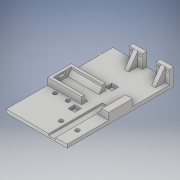
# Autodesk Inventor part: Elevator Slide Top
Saved by Autodesk Inventor 2018 (Build 220112000, 112)
## iProperties
Created: 2017-10-26
Part Number: Elevator Slide Top
Material: Generic
Document SubType Name: Modeling
Designer: thompson.nathaniel
Density: 1 g/cm^3
Appearance: Default
Author: thompson.nathaniel
Autodesk Inventor part; units mm, degrees
ref_plane "YZ Plane" through (0, 0, 0) normal (1, 0, 0) x (0, 1, 0)
ref_plane "XZ Plane" through (0, 0, 0) normal (0, 1, 0) x (-1, 0, 0)
ref_plane "XY Plane" through (0, 0, 0) normal (0, 0, 1) x (1, 0, 0)
sketch "Sketch1" plane through (0, 0, 0) normal (0, 1, 0) x (-1, 0, 0)
  line L0 (0, 0) -> (-114.3, 0)
  line L1 (-114.3, 0) -> (-114.3, 152.4)
  line L2 (-114.3, 152.4) -> (0, 152.4)
  line L3 (0, 152.4) -> (0, 0)
  line L4 (-57.15, 34.925) -> (-69.85, 34.925)
  line L5 (-69.85, 34.925) -> (-69.85, 47.625)
  line L6 (-69.85, 47.625) -> (-57.15, 47.625)
  line L7 (-57.15, 47.625) -> (-57.15, 34.925)
  line L8 (-57.15, 104.775) -> (-69.85, 104.775)
  line L9 (-69.85, 104.775) -> (-69.85, 117.475)
  line L10 (-69.85, 117.475) -> (-57.15, 117.475)
  line L11 (-57.15, 117.475) -> (-57.15, 104.775)
  dimension "d0" = 152.4
  dimension "d1" = 114.3
  dimension "d2" = 12.7
  dimension "d3" = 12.7
  dimension "d4" = 12.7
  dimension "d5" = 12.7
  dimension "d6" = 34.925
  dimension "d7" = 34.925
  dimension "d8" = 44.45
  dimension "d9" = 44.45
  constraints: 24 end point, 6 parallel, 3 horizontal, 3 perpendicular
  measures "d0" distance of L2.end L0.start
  measures "d1" distance of L0.start L0.end
  measures "d2" distance of L4.start L4.end
  measures "d3" distance of L8.start L8.end
  measures "d4" distance of L8.end L9.end
  measures "d5" distance of L4.end L5.end
  measures "d6" distance between parallel lines of L0 L4
  measures "d7" distance between parallel lines of L2 L10
  measures "d8" distance between parallel lines of L1 L5
  measures "d9" distance between parallel lines of L1 L9
extrude "Extrusion1" add sketch "Sketch1" along normal blind 10.16
sketch "Sketch2" plane through (0, 0, 0) normal (-1, 0, 0) x (0, 0, 1)
  line L0 (0, 10.16) -> (152.4, 10.16) projected
  line L1 (53.975, 10.16) -> (98.425, 10.16)
  line L2 (98.425, 10.16) -> (98.425, 22.86)
  line L3 (98.425, 22.86) -> (93.345, 22.86)
  line L4 (93.345, 22.86) -> (93.345, 19.05)
  line L5 (93.345, 19.05) -> (86.614, 10.16)
  line L6 (86.614, 10.16) -> (76.2, 10.16)
  line L7 (65.786, 10.16) -> (59.055, 19.05)
  line L8 (59.055, 19.05) -> (59.055, 22.86)
  line L9 (59.055, 22.86) -> (53.975, 22.86)
  line L10 (53.975, 22.86) -> (53.975, 10.16)
  line L11 (0, 0) -> (0, 10.16) projected
  dimension "d12" = 0
  dimension "d13" = 20.828
  dimension "d14" = 44.45
  dimension "d15" = 3.81
  dimension "d16" = 3.81
  dimension "d17" = 12.7
  dimension "d18" = 12.7
  dimension "d19" = 5.08
  dimension "d20" = 5.08
  dimension "d21" = 11.811
  dimension "d24" = 53.975
  constraints: 20 end point, 5 point on line, 4 perpendicular, 2 vertical, 1 midpoint
  measures "d12" distance from line of L1.start L10
  measures "d13" distance of L5.end L7.start
  measures "d14" distance between parallel lines of L2 L10
  measures "d15" distance of L8.end L7.end
  measures "d16" distance of L3.end L4.end
  measures "d17" distance of L9.end L10.end
  measures "d18" distance of L1.end L2.end
  measures "d19" distance of L8.end L9.end
  measures "d20" distance of L2.end L3.end
  measures "d21" distance from line of L7.start L10
  measures "d24" distance between parallel lines of L11 L10
extrude "Extrusion2" add sketch "Sketch2" against normal blind 63.5
sketch "Sketch4" plane through (0, 10.16, 0) normal (0, 1, 0) x (1, 0, 0)
  circle A0 centre (20.32, -47.625) radius 3.81
  circle A1 centre (44.45, -47.625) radius 3.81
  circle A2 centre (20.32, -104.775) radius 3.81
  circle A3 centre (44.45, -104.775) radius 3.81
  line L0 (0, -53.975) -> (63.5, -53.975) projected
  line L1 (63.5, -98.425) -> (0, -98.425) projected
  line L2 (0, -98.425) -> (0, -152.4) projected
  line L3 (0, 0) -> (0, -53.975) projected
  dimension "d28" = 7.62
  dimension "d29" = 7.62
  dimension "d30" = 7.62
  dimension "d31" = 7.62
  dimension "d32" = 6.35
  dimension "d33" = 6.35
  dimension "d34" = 6.35
  dimension "d35" = 6.35
  dimension "d36" = 20.32
  dimension "d37" = 44.45
  dimension "d38" = 20.32
  dimension "d39" = 44.45
  constraints: 4 centre point
  measures "d28" diameter of A0
  measures "d29" diameter of A1
  measures "d30" diameter of A2
  measures "d31" diameter of A3
  measures "d32" distance from line of L0 A0.centre
  measures "d33" distance from line of L0 A1.centre
  measures "d34" distance from line of L1 A3.centre
  measures "d35" distance from line of L1 A2.centre
  measures "d36" distance from line of L2 A2.centre
  measures "d37" distance from line of L2 A3.centre
  measures "d38" distance from line of L3 A0.centre
  measures "d39" distance from line of L3 A1.centre
extrude "Extrusion4" cut sketch "Sketch4" against normal blind 10.16
sketch "Sketch5" plane through (0, 0, 152.4) normal (0, 0, 1) x (1, 0, 0)
  line L0 (0, 0) -> (114.3, 0) projected
  line L1 (0, 10.16) -> (114.3, 10.16)
  line L2 (114.3, 10.16) -> (114.3, 0)
  line L3 (114.3, 0) -> (0, 0)
  line L4 (0, 0) -> (0, 10.16)
  constraints: 8 end point, 2 parallel, 1 horizontal, 1 perpendicular
extrude "Extrusion5" add sketch "Sketch5" along normal blind 25.4
sketch "Sketch6" plane through (114.3, 0, 0) normal (0, 0, -1) x (-1, 0, 0)
  line L0 (0, 10.16) -> (114.3, 10.16) projected
  line L1 (114.3, 0) -> (0, 0) projected
  line L2 (0, 10.16) -> (114.3, 10.16)
  line L3 (114.3, 10.16) -> (114.3, 0)
  line L4 (114.3, 0) -> (0, 0)
  line L5 (0, 0) -> (0, 10.16)
  constraints: 8 end point, 2 parallel, 1 horizontal, 1 perpendicular
extrude "Extrusion6" add sketch "Sketch6" along normal blind 25.4
sketch "Sketch7" plane through (0, 10.16, 0) normal (0, 1, 0) x (1, 0, 0)
  line L0 (114.3, 25.4) -> (114.3, -177.8) projected
  line L1 (114.3, -98.425) -> (101.6, -98.425)
  line L2 (101.6, -98.425) -> (101.6, -53.975)
  line L3 (101.6, -53.975) -> (114.3, -53.975)
  line L4 (114.3, -53.975) -> (114.3, -98.425)
  line L5 (0, -98.425) -> (63.5, -98.425) projected
  line L6 (0, -53.975) -> (63.5, -53.975) projected
  point P0 (0, 0)
  dimension "d46" = 0
  dimension "d47" = 0
  dimension "d48" = 12.7
  constraints: 8 end point, 2 parallel, 1 horizontal, 1 perpendicular, 1 point on line
  measures "d46" distance between parallel lines of L1 L5
  measures "d47" distance between parallel lines of L3 L6
  measures "d48" distance between parallel lines of L0 L2
extrude "Extrusion7" add sketch "Sketch7" along normal blind 12.7
sketch "Sketch8" plane through (0, 10.16, 0) normal (0, 1, 0) x (1, 0, 0)
  line L0 (114.3, -177.8) -> (0, -177.8) projected
  line L1 (80.01, -177.8) -> (92.71, -177.8)
  line L2 (92.71, -177.8) -> (92.71, -76.2)
  line L3 (92.71, -76.2) -> (80.01, -76.2)
  line L4 (80.01, -76.2) -> (80.01, -177.8)
  line L5 (101.6, -98.425) -> (101.6, -53.975) projected
  point P0 (0, 0)
  dimension "d51" = 8.89
  dimension "d52" = 12.7
  dimension "d53" = 101.6
  constraints: 8 end point, 2 parallel, 1 horizontal, 1 perpendicular, 1 point on line
  measures "d51" distance between parallel lines of L5 L2
  measures "d52" distance between parallel lines of L4 L2
  measures "d53" distance between parallel lines of L0 L3
extrude "Extrusion8" cut sketch "Sketch8" against normal blind 3.175
sketch "Sketch9" plane through (0, 0, 0) normal (0, -1, 0) x (1, 0, 0)
  line L0 (0, 177.8) -> (0, -25.4) projected
  line L1 (114.3, 177.8) -> (92.71, 177.8) projected
  line L2 (0, -25.4) -> (114.3, -25.4)
  line L3 (114.3, -25.4) -> (114.3, 177.8)
  line L4 (114.3, 177.8) -> (0, 177.8)
  line L5 (0, 177.8) -> (0, -25.4)
  point P0 (0, 0)
  constraints: 8 end point, 2 parallel, 1 horizontal, 1 perpendicular
extrude "Extrusion9" cut sketch "Sketch9" against normal blind 3.81
sketch "Sketch10" plane through (0, 10.16, 0) normal (0, 1, 0) x (1, 0, 0)
  circle A0 centre (71.12, -144.145) radius 3.81
  circle A1 centre (101.6, -144.145) radius 3.81
  line L0 (0, -93.345) -> (63.5, -93.345) projected
  line L1 (92.71, -76.2) -> (92.71, -177.8) projected
  line L2 (80.01, -177.8) -> (80.01, -76.2) projected
  point P0 (0, 0)
  dimension "d58" = 50.8
  dimension "d59" = 50.8
  dimension "d60" = 7.62
  dimension "d61" = 7.62
  dimension "d68" = 8.89
  dimension "d69" = 8.89
  constraints: 2 centre point
  measures "d58" distance from line of L0 A0.centre
  measures "d59" distance from line of L0 A1.centre
  measures "d60" diameter of A1
  measures "d61" diameter of A0
  measures "d68" distance from line of L1 A1.centre
  measures "d69" distance from line of L2 A0.centre
extrude "Extrusion10" cut sketch "Sketch10" against normal blind 25.4
sketch "Sketch11" plane through (0, 0, 177.8) normal (0, 0, 1) x (1, 0, 0)
  line L0 (0, 10.16) -> (0, 19.05) projected
  line L1 (0, 10.16) -> (114.3, 10.16)
  line L2 (114.3, 10.16) -> (114.3, 3.81)
  line L3 (114.3, 3.81) -> (0, 3.81)
  line L4 (0, 3.81) -> (0, 10.16)
  point P0 (0, 0)
  constraints: 8 end point, 2 parallel, 1 horizontal, 1 perpendicular
extrude "Extrusion11" cut sketch "Sketch11" against normal blind 1.397
sketch "Sketch12" plane through (114.3, 0, -25.4) normal (0, 0, -1) x (-1, 0, 0)
  line L0 (114.3, 19.05) -> (114.3, 10.16) projected
  line L1 (0, 10.16) -> (0, 3.81) projected
  line L2 (114.3, 10.16) -> (0, 10.16)
  line L3 (0, 10.16) -> (0, 3.81)
  line L4 (0, 3.81) -> (114.3, 3.81)
  line L5 (114.3, 3.81) -> (114.3, 10.16)
  point P0 (114.3, 0)
  constraints: 8 end point, 2 parallel, 1 horizontal, 1 perpendicular
extrude "Extrusion12" cut sketch "Sketch12" against normal blind 1.397
sketch "Sketch13" plane through (0, 22.86, 59.055) normal (0, 1, 0) x (1, 0, 0)
  line L0 (0, 0) -> (63.5, 0) projected
  line L1 (0, -34.29) -> (63.5, -34.29) projected
  line L2 (0, 0) -> (4.953, 0)
  line L3 (4.953, 0) -> (4.953, -34.29)
  line L4 (4.953, -34.29) -> (0, -34.29)
  line L5 (0, -34.29) -> (0, 0)
  point P0 (0, 59.055)
  dimension "d70" = 4.953
  constraints: 8 end point, 2 parallel, 1 horizontal, 1 perpendicular, 1 point on line
  measures "d70" distance between parallel lines of L3 L5
extrude "Extrusion13" add sketch "Sketch13" against normal blind 12.7
sketch "Sketch14" plane through (4.953, 22.86, 93.345) normal (1, 0, 0) x (0, 0, -1)
  line L0 (11.176, -2.032) -> (23.114, -2.032)
  line L1 (23.114, -2.032) -> (23.114, -7.62)
  line L2 (23.114, -7.62) -> (11.176, -7.62)
  line L3 (11.176, -7.62) -> (11.176, -2.032)
  line L4 (27.559, -12.7) -> (6.731, -12.7) projected
  point P0 (93.345, -22.86)
  dimension "d73" = 5.08
  dimension "d74" = 5.588
  dimension "d75" = 4.445
  dimension "d76" = 4.445
  constraints: 8 end point, 2 parallel, 1 horizontal, 1 perpendicular
  measures "d73" distance between parallel lines of L4 L2
  measures "d74" distance of L0.end L1.end
  measures "d75" distance from line of L4.end L3
  measures "d76" distance from line of L4.start L1
extrude "Extrusion14" cut sketch "Sketch14" against normal blind 12.7
sketch "Sketch15" plane through (0, 10.16, 0) normal (0, 1, 0) x (1, 0, 0)
  line L0 (101.6, -98.425) -> (92.71, -98.425)
  line L1 (92.71, -98.425) -> (92.71, -53.975)
  line L2 (92.71, -53.975) -> (101.6, -53.975)
  line L3 (101.6, -53.975) -> (101.6, -98.425)
  line L4 (101.6, -53.975) -> (114.3, -53.975) projected
  line L5 (92.71, -76.2) -> (92.71, -176.403) projected
  point P0 (0, 0)
  dimension "d79" = 0
  dimension "d80" = 0
  constraints: 8 end point, 2 parallel, 1 horizontal, 1 perpendicular
  measures "d79" distance between parallel lines of L4 L2
  measures "d80" distance between parallel lines of L5 L1
extrude "Extrusion15" add sketch "Sketch15" along normal blind 9.9568
chamfer "Chamfer1" distance 8.89 angle 45 1 edges at (92.71, 20.1168, 76.2)
sketch "Sketch16" plane through (0, 10.16, 0) normal (0, 1, 0) x (1, 0, 0)
  point P0 (0, 0)
sketch "Sketch17" plane through (0, 10.16, 0) normal (0, 1, 0) x (1, 0, 0)
  line L0 (114.3, 24.003) -> (0, 24.003) projected
  line L1 (114.3, 24.003) -> (114.3, 16.383)
  line L2 (114.3, -176.403) -> (114.3, 24.003) projected
  line L3 (105.41, 16.383) -> (105.41, -1.397)
  line L4 (105.41, -1.397) -> (97.79, -1.397)
  line L5 (97.79, -1.397) -> (97.79, 16.383)
  line L6 (97.79, 16.383) -> (88.9, 16.383)
  line L7 (88.9, 16.383) -> (88.9, 24.003)
  line L8 (88.9, 24.003) -> (114.3, 24.003)
  line L9 (63.5, 24.003) -> (63.5, 16.383)
  line L10 (63.5, 16.383) -> (54.61, 16.383)
  line L11 (54.61, 16.383) -> (54.61, -1.397)
  line L12 (54.61, -1.397) -> (46.99, -1.397)
  line L13 (46.99, -1.397) -> (46.99, 16.383)
  line L14 (46.99, 16.383) -> (38.1, 16.383)
  line L15 (38.1, 16.383) -> (38.1, 24.003)
  line L16 (38.1, 24.003) -> (63.5, 24.003)
  line L17 (105.41, 16.383) -> (114.3, 16.383)
  point P0 (0, 0)
  dimension "d86" = 25.4
  dimension "d87" = 8.89
  dimension "d88" = 7.62
  dimension "d89" = 17.78
  dimension "d90" = 17.78
  dimension "d91" = 7.62
  dimension "d92" = 8.89
  dimension "d93" = 25.4
  dimension "d94" = 7.62
  dimension "d95" = 25.4
  constraints: 32 end point, 10 perpendicular, 9 point on line, 1 horizontal, 1 vertical
  measures "d86" distance of L7.end L0.start
  measures "d87" distance of L3.start L1.end
  measures "d88" distance of L3.end L4.end
  measures "d89" distance of L3.start L3.end
  measures "d90" distance of L10.end L11.end
  measures "d91" distance of L11.end L12.end
  measures "d92" distance between parallel lines of L9 L11
  measures "d93" distance between parallel lines of L9 L15
  measures "d94" distance between parallel lines of L0 L10
  measures "d95" distance between parallel lines of L7 L9
extrude "Extrusion16" add sketch "Sketch17" along normal blind 25.4
chamfer "Chamfer2" distance 17.78 distance2 25.4 1 edges at (101.6, 35.56, 1.397) measured on face at (101.6, 35.56, 0.897)
chamfer "Chamfer3" distance 17.78 distance2 25.4 1 edges at (50.8, 35.56, 1.397) measured on face at (50.8, 35.56, 0.897)
sketch "Sketch18" plane through (54.61, 10.16, -16.383) normal (0, 0, 1) x (1, 0, 0)
  circle A0 centre (-11.43, 20.32) radius 2.54
  circle A1 centre (3.81, 20.32) radius 2.54
  circle A2 centre (39.37, 20.32) radius 2.54
  circle A3 centre (54.61, 20.32) radius 2.54
  line L0 (34.29, 0) -> (34.29, 25.4) projected
  line L1 (59.69, 0) -> (59.69, 25.4) projected
  line L2 (50.8, 25.4) -> (59.69, 25.4) projected
  line L3 (34.29, 25.4) -> (43.18, 25.4) projected
  line L4 (8.89, 0) -> (8.89, 25.4) projected
  line L5 (-16.51, 0) -> (-16.51, 25.4) projected
  line L6 (0, 25.4) -> (8.89, 25.4) projected
  line L7 (-16.51, 25.4) -> (-7.62, 25.4) projected
  point P0 (-54.61, -10.16)
  dimension "d104" = 5.08
  dimension "d105" = 5.08
  dimension "d106" = 5.08
  dimension "d107" = 5.08
  dimension "d108" = 5.08
  dimension "d109" = 5.08
  dimension "d110" = 5.08
  dimension "d111" = 5.08
  dimension "d112" = 5.08
  dimension "d113" = 5.08
  dimension "d114" = 5.08
  dimension "d115" = 5.08
  constraints: 4 centre point
  measures "d104" diameter of A0
  measures "d105" diameter of A1
  measures "d106" distance from line of L0 A2.centre
  measures "d107" distance from line of L1 A3.centre
  measures "d108" distance from line of L2 A3.centre
  measures "d109" distance from line of L3 A2.centre
  measures "d110" distance from line of L4 A1.centre
  measures "d111" distance from line of L5 A0.centre
  measures "d112" distance from line of L6 A1.centre
  measures "d113" distance from line of L7 A0.centre
  measures "d114" diameter of A2
  measures "d115" diameter of A3
extrude "Extrusion17" cut sketch "Sketch18" against normal blind 25.4
body "Solid1"
